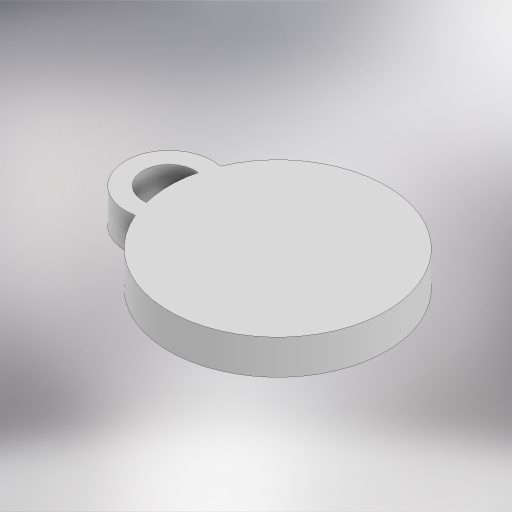
# Autodesk Inventor part: keyring
Saved by Autodesk Inventor 2024.3 (Build 283343000, 343)
## iProperties
Created: 2025-07-28
Part Number: keyring
Material: Generic
Document SubType Name: Modeling
Designer: danie
Density: 1 g/cm^3
Appearance: Default
Author: danie
Autodesk Inventor part; units mm, degrees
ref_plane "YZ Plane" through (0, 0, 0) normal (1, 0, 0) x (0, 1, 0)
ref_plane "XZ Plane" through (0, 0, 0) normal (0, 1, 0) x (-1, 0, 0)
ref_plane "XY Plane" through (0, 0, 0) normal (0, 0, 1) x (1, 0, 0)
sketch "Sketch1" plane through (0, 0, 0) normal (0, 1, 0) x (-1, 0, 0)
  circle A0 centre (0, 0) radius 12.5
  circle A1 centre (12.5, 0) radius 5
  circle A2 centre (12.5, 0) radius 3
  point P0 (12.14, 2.9783)
  point P1 (12.14, -2.9783)
  point P2 (11.5, -4.899)
  point P3 (11.5, 4.899)
  dimension "d0" = 25
  dimension "d3" = 10
  dimension "d4" = 2
  constraints: 2 centre point, 2 coincident, 3 other
  measures "d3" diameter of A1
  measures "d4" radial gap between concentric circles of A1 A2
extrude "Extrusion1" add sketch "Sketch1" along normal blind 4 contours A0 A2 | A2 A0 A1 | A0 A1 A2 | A1 A0 picked at (11.5157, -0.5732)
body "Solid1"
